# Autodesk Inventor part: TUSB2046BIRHBIRHB
Saved by Autodesk Inventor 2016 SP1 (Build 200210100, 210)
## iProperties
Created: 2015-11-24
Part Number: TUSB2046BIRHBIRHB
Material: Generic
Document SubType Name: Modeling
Designer: PhillipD
Density: 1 g/cm^3
Appearance: RHB_S-PQFP-N32, TUSB2046BIRHBIRHB
Author: PhillipD
Autodesk Inventor part; units mm, degrees
ref_plane "YZ Plane" through (0, 0, 0) normal (1, 0, 0) x (0, 1, 0)
ref_plane "XZ Plane" through (0, 0, 0) normal (0, 1, 0) x (-1, 0, 0)
ref_plane "XY Plane" through (0, 0, 0) normal (0, 0, 1) x (1, 0, 0)
sketch "RHB_S-PQFP-N32, TUSB2046BIRHBIRHB_49" plane through (0, 0, 0) normal (0, 0, 1) x (1, 0, 0)
  line L0 (-3.3274, 3.0734) -> (2.65, 3.0734)
  line L1 (2.65, 3.0734) -> (2.65, -2.65)
  line L2 (2.65, -2.65) -> (-3.3274, -2.65)
  line L3 (-3.3274, -2.65) -> (-3.3274, 3.0734)
  constraints: 8 end point
extrude "Extrusion1" add sketch "RHB_S-PQFP-N32, TUSB2046BIRHBIRHB_49" along normal blind 1
body "Solid1"
